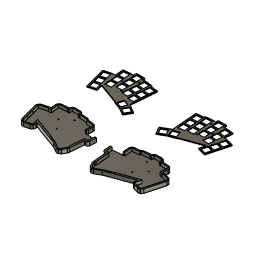
Architeuthis Dux v2 (Autodesk Fusion 360 design; units mm, degrees)
Autodesk Fusion 360 part; units mm, degrees
note: some values were not read from the file. Set by a fixed rule: which sketch regions a step uses.
sketch "Sketch1" plane through (0, 0, 0) normal (0, 0, 1) x (1, 0, 0)
  line L0 (25.9385, -60.9067) -> (30.3403, -77.3278)
  line L1 (30.3403, -77.3278) -> (12.954, -81.9861)
  line L2 (12.954, -81.9861) -> (8.5522, -65.565)
  line L3 (21.5392, -44.4856) -> (25.9385, -60.9067)
  line L4 (25.9385, -60.9067) -> (8.5522, -65.565)
  line L5 (25.9385, -60.9067) -> (8.5522, -65.565)
  line L6 (8.5522, -65.565) -> (4.1529, -49.1439)
  line L7 (4.1529, -49.1439) -> (21.5392, -44.4856)
  line L8 (-0.2438, -32.7228) -> (17.1399, -28.0645)
  line L9 (17.1399, -28.0645) -> (21.5392, -44.4856)
  line L10 (4.1529, -49.1439) -> (-0.2438, -32.7228)
  line L11 (43.5762, -40.5994) -> (45.0571, -57.5361)
  line L12 (45.0571, -57.5361) -> (27.1272, -59.1033)
  line L13 (27.1272, -59.1033) -> (25.6438, -42.1691)
  line L14 (25.6438, -42.1691) -> (43.5762, -40.5994)
  line L15 (43.5762, -40.5994) -> (25.6438, -42.1691)
  line L16 (43.5762, -40.5994) -> (25.6438, -42.1691)
  line L17 (25.6438, -42.1691) -> (24.163, -25.2349)
  line L18 (24.163, -25.2349) -> (42.0954, -23.6652)
  line L19 (42.0954, -23.6652) -> (43.5762, -40.5994)
  line L20 (24.163, -25.2349) -> (22.6822, -8.2982)
  line L21 (22.6822, -8.2982) -> (40.6121, -6.7285)
  line L22 (40.6121, -6.7285) -> (42.0954, -23.6652)
  line L23 (45.4711, -34.0741) -> (63.4695, -34.0741)
  line L24 (63.4695, -34.0741) -> (63.4695, -51.0743)
  line L25 (63.4695, -51.0743) -> (45.4711, -51.0743)
  line L26 (45.4711, -51.0743) -> (45.4711, -34.0741)
  line L27 (45.4711, -34.0741) -> (63.4695, -34.0741)
  line L28 (45.4711, -17.0739) -> (63.4695, -17.0739)
  line L29 (45.4711, -34.0741) -> (45.4711, -17.0739)
  line L30 (63.4695, -34.0741) -> (45.4711, -34.0741)
  line L31 (63.4695, -17.0739) -> (63.4695, -34.0741)
  line L32 (63.4695, -0.0737) -> (63.4695, -17.0739)
  line L33 (45.4711, -17.0739) -> (45.4711, -0.0737)
  line L34 (45.4711, -0.0737) -> (63.4695, -0.0737)
  line L35 (65.5269, -39.0525) -> (83.4593, -40.6222)
  line L36 (83.4593, -40.6222) -> (81.976, -57.5564)
  line L37 (81.976, -57.5564) -> (64.0461, -55.9892)
  line L38 (64.0461, -55.9892) -> (65.5269, -39.0525)
  line L39 (65.5269, -39.0525) -> (83.4593, -40.6222)
  line L40 (67.0077, -22.1183) -> (84.9401, -23.6855)
  line L41 (65.5269, -39.0525) -> (67.0077, -22.1183)
  line L42 (86.421, -6.7513) -> (84.9401, -23.6855)
  line L43 (67.0077, -22.1183) -> (68.4911, -5.1816)
  line L44 (68.4911, -5.1816) -> (86.421, -6.7513)
  line L45 (83.2129, -43.4442) -> (101.1428, -45.0139)
  line L46 (101.1428, -45.0139) -> (99.662, -61.9481)
  line L47 (99.662, -61.9481) -> (81.7296, -60.3809)
  line L48 (81.7296, -60.3809) -> (83.2129, -43.4442)
  line L49 (83.2129, -43.4442) -> (101.1428, -45.0139)
  line L50 (84.6938, -26.51) -> (102.6262, -28.0772)
  line L51 (102.6262, -28.0772) -> (101.1428, -45.0139)
  line L52 (86.1746, -9.5733) -> (104.107, -11.143)
  line L53 (102.6262, -28.0772) -> (84.6938, -26.51)
  line L54 (104.107, -11.143) -> (102.6262, -28.0772)
  line L55 (83.7946, -65.5396) -> (100.7085, -71.6966)
  line L56 (94.8944, -87.6706) -> (77.9805, -81.5137)
  line L57 (77.9805, -81.5137) -> (83.7946, -65.5396)
  line L58 (100.7085, -71.6966) -> (94.8944, -87.6706)
  line L59 (103.5533, -73.0225) -> (119.1412, -82.0217)
  line L60 (119.1412, -82.0217) -> (110.6424, -96.7435)
  line L61 (110.6424, -96.7435) -> (95.0519, -87.7443)
  line L62 (95.0519, -87.7443) -> (103.5533, -73.0225)
  line L63 (116.5835, -26.9875) -> (116.1415, -32.0472)
  line L64 (108.9914, -26.322) -> (116.5835, -26.9875)
  line L65 (108.5494, -31.3817) -> (108.9914, -26.322)
  line L66 (116.1415, -32.0472) -> (108.5494, -31.3817)
  line L67 (128.7755, -30.3657) -> (123.1951, -29.878)
  line L68 (123.0224, -31.8694) -> (123.1951, -29.878)
  line L69 (128.6002, -32.3571) -> (128.7755, -30.3657)
  line L70 (122.7734, -31.8491) -> (121.7193, -43.9014)
  line L71 (128.8491, -32.3799) -> (127.795, -44.4348)
  line L72 (127.795, -44.4348) -> (121.7193, -43.9014)
  line L73 (128.8491, -32.3799) -> (122.7734, -31.8491)
  arc A0 (94.8962, -87.6719) -> (95.0542, -87.7456) centre (94.5542, -88.6116) cw
  line L74 (83.4593, -40.6222) -> (84.9401, -23.6855)
  line L75 (84.6938, -26.51) -> (86.1746, -9.5733)
  line L76 (83.2129, -43.4442) -> (84.6938, -26.51)
  line L77 (2.0726, -33.655) -> (5.6972, -47.178)
  line L78 (5.6972, -47.178) -> (19.2202, -43.5559)
  line L79 (19.2202, -43.5559) -> (15.5956, -30.033)
  line L80 (15.5956, -30.033) -> (2.0726, -33.655)
  line L81 (6.4719, -50.0761) -> (10.0965, -63.5991)
  line L82 (10.0965, -63.5991) -> (23.6195, -59.9745)
  line L83 (23.6195, -59.9745) -> (19.9949, -46.4515)
  line L84 (19.9949, -46.4515) -> (6.4719, -50.0761)
  line L85 (10.8737, -66.4972) -> (14.4958, -80.0202)
  line L86 (14.4958, -80.0202) -> (28.0187, -76.3956)
  line L87 (28.0187, -76.3956) -> (24.3967, -62.8726)
  line L88 (24.3967, -62.8726) -> (10.8737, -66.4972)
  line L89 (27.7673, -43.4899) -> (28.989, -57.437)
  line L90 (28.989, -57.437) -> (42.9336, -56.2153)
  line L91 (42.9336, -56.2153) -> (41.7144, -42.2681)
  line L92 (41.7144, -42.2681) -> (27.7673, -43.4899)
  line L93 (26.2865, -26.5532) -> (27.5057, -40.5003)
  line L94 (27.5057, -40.5003) -> (41.4528, -39.2811)
  line L95 (41.4528, -39.2811) -> (40.2336, -25.334)
  line L96 (40.2336, -25.334) -> (26.2865, -26.5532)
  line L97 (24.8056, -9.619) -> (26.0248, -23.5661)
  line L98 (26.0248, -23.5661) -> (39.972, -22.3444)
  line L99 (39.972, -22.3444) -> (38.7502, -8.3972)
  line L100 (38.7502, -8.3972) -> (24.8056, -9.619)
  line L101 (47.4701, -1.5748) -> (47.4701, -15.5727)
  line L102 (47.4701, -15.5727) -> (61.4705, -15.5727)
  line L103 (61.4705, -15.5727) -> (61.4705, -1.5748)
  line L104 (61.4705, -1.5748) -> (47.4701, -1.5748)
  line L105 (47.4701, -18.5725) -> (47.4701, -32.573)
  line L106 (47.4701, -32.573) -> (61.4705, -32.573)
  line L107 (61.4705, -32.573) -> (61.4705, -18.5725)
  line L108 (61.4705, -18.5725) -> (47.4701, -18.5725)
  line L109 (47.4701, -35.5727) -> (47.4701, -49.5732)
  line L110 (47.4701, -49.5732) -> (61.4705, -49.5732)
  line L111 (61.4705, -49.5732) -> (61.4705, -35.5727)
  line L112 (61.4705, -35.5727) -> (47.4701, -35.5727)
  line L113 (67.3887, -40.7213) -> (66.1695, -54.6684)
  line L114 (66.1695, -54.6684) -> (80.1141, -55.8876)
  line L115 (80.1141, -55.8876) -> (81.3359, -41.943)
  line L116 (81.3359, -41.943) -> (67.3887, -40.7213)
  line L117 (68.8696, -23.7871) -> (67.6504, -37.7342)
  line L118 (67.6504, -37.7342) -> (81.5975, -38.9534)
  line L119 (81.5975, -38.9534) -> (82.8167, -25.0063)
  line L120 (82.8167, -25.0063) -> (68.8696, -23.7871)
  line L121 (70.3529, -6.8504) -> (69.1312, -20.7975)
  line L122 (69.1312, -20.7975) -> (83.0783, -22.0167)
  line L123 (83.0783, -22.0167) -> (84.3001, -8.0721)
  line L124 (84.3001, -8.0721) -> (70.3529, -6.8504)
  line L125 (88.0364, -11.242) -> (86.8172, -25.1892)
  line L126 (86.8172, -25.1892) -> (100.7643, -26.4084)
  line L127 (100.7643, -26.4084) -> (101.9835, -12.4638)
  line L128 (101.9835, -12.4638) -> (88.0364, -11.242)
  line L129 (86.5556, -28.1788) -> (85.3338, -42.1234)
  line L130 (85.3338, -42.1234) -> (99.281, -43.3451)
  line L131 (99.281, -43.3451) -> (100.5027, -29.398)
  line L132 (100.5027, -29.398) -> (86.5556, -28.1788)
  line L133 (85.0722, -45.1129) -> (83.853, -59.0601)
  line L134 (83.853, -59.0601) -> (97.8002, -60.2793)
  line L135 (97.8002, -60.2793) -> (99.0194, -46.3321)
  line L136 (99.0194, -46.3321) -> (85.0722, -45.1129)
  line L137 (85.1611, -67.6326) -> (80.3732, -80.7898)
  line L138 (80.3732, -80.7898) -> (93.5279, -85.5777)
  line L139 (93.5279, -85.5777) -> (98.3158, -72.4205)
  line L140 (98.3158, -72.4205) -> (85.1611, -67.6326)
  line L141 (104.5337, -75.3212) -> (97.536, -87.4446)
  line L142 (97.536, -87.4446) -> (109.6594, -94.4448)
  line L143 (109.6594, -94.4448) -> (116.6597, -82.3214)
  line L144 (116.6597, -82.3214) -> (104.5337, -75.3212)
  line L145 (3.1869, -49.4026) -> (-1.4684, -32.0157)
  line L146 (-1.4684, -32.0157) -> (17.8471, -26.8397)
  line L147 (17.8471, -26.8397) -> (22.5051, -44.2268)
  line L148 (22.5051, -44.2268) -> (26.9044, -60.6478)
  line L149 (26.9044, -60.6478) -> (31.5651, -78.0349)
  line L150 (31.5651, -78.0349) -> (12.247, -83.2108)
  line L151 (12.247, -83.2108) -> (7.5863, -65.8239)
  line L152 (7.5863, -65.8239) -> (3.1869, -49.4026)
  line L153 (23.2539, -26.3183) -> (21.5989, -7.3892)
  line L154 (21.5989, -7.3892) -> (41.521, -5.6451)
  line L155 (41.521, -5.6451) -> (43.1789, -24.5742)
  line L156 (23.2539, -26.3183) -> (43.1789, -24.5742)
  line L157 (44.4711, -18.0739) -> (44.4711, 0.9263)
  line L158 (44.4711, 0.9263) -> (64.4695, 0.9263)
  line L159 (64.4695, 0.9263) -> (64.4695, -18.0739)
  line L160 (44.4711, -18.0739) -> (64.4695, -18.0739)
  line L161 (65.9243, -23.0274) -> (67.5822, -4.0982)
  line L162 (67.5822, -4.0982) -> (87.5043, -5.8423)
  line L163 (87.5043, -5.8423) -> (85.8492, -24.7688)
  line L164 (65.9243, -23.0274) -> (85.8492, -24.7688)
  line L165 (83.6105, -27.4191) -> (85.2655, -8.4899)
  line L166 (85.2655, -8.4899) -> (105.1903, -10.234)
  line L167 (105.1903, -10.234) -> (103.5352, -29.1604)
  line L168 (103.5352, -29.1604) -> (83.6105, -27.4191)
  line L169 (76.6988, -82.1113) -> (83.1969, -64.2579)
  line L170 (83.1969, -64.2579) -> (101.9902, -71.0989)
  line L171 (101.9902, -71.0989) -> (95.4921, -88.9524)
  line L172 (95.4921, -88.9524) -> (76.6988, -82.1113)
  line L173 (120.5072, -81.6556) -> (111.0085, -98.1095)
  line L174 (111.0085, -98.1095) -> (93.6857, -88.1104)
  line L175 (93.6857, -88.1104) -> (103.1873, -71.6565)
  line L176 (103.1873, -71.6565) -> (120.5072, -81.6556)
  point P0 (104.5337, -75.3212)
  point P1 (97.536, -87.4446)
  point P2 (109.6594, -94.4448)
  point P3 (116.6597, -82.3214)
  point P4 (93.5279, -85.5777)
  point P5 (98.3158, -72.4205)
  point P6 (85.1611, -67.6326)
  point P7 (80.3732, -80.7898)
  point P8 (97.8002, -60.2793)
  point P9 (99.0194, -46.3321)
  point P10 (85.0722, -45.1129)
  point P11 (83.853, -59.0601)
  point P12 (85.3338, -42.1234)
  point P13 (99.281, -43.3451)
  point P14 (100.5027, -29.398)
  point P15 (86.5556, -28.1788)
  point P16 (86.8172, -25.1892)
  point P17 (88.0364, -11.242)
  point P18 (101.9835, -12.4638)
  point P19 (100.7643, -26.4084)
  point P20 (83.0783, -22.0167)
  point P21 (84.3001, -8.0721)
  point P22 (70.3529, -6.8504)
  point P23 (69.1312, -20.7975)
  point P24 (68.8696, -23.7871)
  point P25 (82.8167, -25.0063)
  point P26 (81.5975, -38.9534)
  point P27 (67.6504, -37.7342)
  point P28 (67.3887, -40.7213)
  point P29 (81.3359, -41.943)
  point P30 (80.1141, -55.8876)
  point P31 (66.1695, -54.6684)
  point P32 (61.4705, -49.5732)
  point P33 (61.4705, -35.5727)
  point P34 (47.4701, -35.5727)
  point P35 (47.4701, -49.5732)
  point P36 (47.4701, -32.573)
  point P37 (61.4705, -32.573)
  point P38 (61.4705, -18.5725)
  point P39 (47.4701, -18.5725)
  point P40 (47.4701, -15.5727)
  point P41 (61.4705, -15.5727)
  point P42 (61.4705, -1.5748)
  point P43 (47.4701, -1.5748)
  point P44 (38.7502, -8.3972)
  point P45 (24.8056, -9.619)
  point P46 (26.0248, -23.5661)
  point P47 (39.972, -22.3444)
  point P48 (40.2336, -25.334)
  point P49 (26.2865, -26.5532)
  point P50 (41.4528, -39.2811)
  point P51 (27.5057, -40.5003)
  point P52 (27.7673, -43.4899)
  point P53 (41.7144, -42.2681)
  point P54 (42.9336, -56.2153)
  point P55 (28.989, -57.437)
  point P56 (15.5956, -30.033)
  point P57 (2.0726, -33.655)
  point P58 (19.2202, -43.5559)
  point P59 (5.6972, -47.178)
  point P60 (6.4719, -50.0761)
  point P61 (19.9949, -46.4515)
  point P62 (23.6195, -59.9745)
  point P63 (10.0965, -63.5991)
  point P64 (24.3967, -62.8726)
  point P65 (28.0187, -76.3956)
  point P66 (14.4958, -80.0202)
  point P67 (10.8737, -66.4972)
  dimension "d8" = -1
  dimension "d9" = 1
  dimension "d10" = 1
  dimension "d11" = 1
  dimension "d12" = -1
  dimension "d13" = -1
  dimension "d14" = -1
  constraint coincident P57 L77.start
  constraint coincident P59 L77.end
  constraint coincident P58 L78.end
  constraint coincident P56 L79.end
  constraint parallel L77 L79
  constraint parallel L78 L80
  constraint coincident P60 L81.start
  constraint coincident P63 L81.end
  constraint parallel L77 L81
  constraint coincident P62 L82.end
  constraint perpendicular L81 L82
  constraint coincident P61 L83.end
  constraint parallel L81 L83
  constraint perpendicular L81 L84
  constraint coincident P67 L85.start
  constraint coincident P66 L85.end
  constraint coincident P65 L86.end
  constraint parallel L82 L86
  constraint coincident P64 L87.end
  constraint parallel L85 L87
  constraint coincident P52 L89.start
  constraint coincident P55 L89.end
  constraint coincident P54 L90.end
  constraint coincident P53 L91.end
  constraint perpendicular L89 L92
  constraint coincident P49 L93.start
  constraint coincident P51 L93.end
  constraint coincident P50 L94.end
  constraint coincident P48 L95.end
  constraint coincident P45 L97.start
  constraint coincident P46 L97.end
  constraint parallel L93 L97
  constraint coincident P47 L98.end
  constraint coincident P44 L99.end
  constraint perpendicular L98 L99
  constraint coincident P43 L101.start
  constraint coincident P40 L101.end
  constraint parallel L33 L101
  constraint coincident P41 L102.end
  constraint perpendicular L101 L102
  constraint coincident P42 L103.end
  constraint perpendicular L102 L103
  constraint perpendicular L101 L104
  constraint coincident P39 L105.start
  constraint coincident P36 L105.end
  constraint perpendicular L28 L105
  constraint coincident P37 L106.end
  constraint perpendicular L105 L106
  constraint coincident P38 L107.end
  constraint perpendicular L106 L107
  constraint perpendicular L107 L108
  constraint coincident P34 L109.start
  constraint coincident P35 L109.end
  constraint perpendicular L106 L109
  constraint coincident P32 L110.end
  constraint perpendicular L109 L110
  constraint coincident P33 L111.end
  constraint perpendicular L106 L111
  constraint perpendicular L109 L112
  constraint coincident P28 L113.start
  constraint coincident P31 L113.end
  constraint coincident P30 L114.end
  constraint coincident P29 L115.end
  constraint coincident P24 L117.start
  constraint coincident P27 L117.end
  constraint coincident P26 L118.end
  constraint perpendicular L117 L118
  constraint coincident P25 L119.end
  constraint perpendicular L118 L119
  constraint perpendicular L117 L120
  constraint coincident P22 L121.start
  constraint coincident P23 L121.end
  constraint coincident P20 L122.end
  constraint coincident P21 L123.end
  constraint coincident P17 L125.start
  constraint coincident P16 L125.end
  constraint coincident P19 L126.end
  constraint perpendicular L125 L126
  constraint coincident P18 L127.end
  constraint coincident P15 L129.start
  constraint coincident P12 L129.end
  constraint coincident P13 L130.end
  constraint parallel L128 L130
  constraint coincident P14 L131.end
  constraint perpendicular L130 L131
  constraint coincident P10 L133.start
  constraint coincident P11 L133.end
  constraint coincident P8 L134.end
  constraint perpendicular L133 L134
  constraint coincident P9 L135.end
  constraint perpendicular L134 L135
  constraint perpendicular L135 L136
  constraint coincident P6 L137.start
  constraint coincident P7 L137.end
  constraint coincident P4 L138.end
  constraint coincident P5 L139.end
  constraint parallel L137 L139
  constraint parallel L138 L140
  constraint coincident P0 L141.start
  constraint coincident P1 L141.end
  constraint coincident P2 L142.end
  constraint coincident P3 L143.end
  constraint perpendicular L142 L143
sketch "Sketch2" plane through (0, 0, 0) normal (0, 0, 1) x (1, 0, 0)
  arc A0 (12.963, -80.5576) -> (11.5653, -78.7359) centre (14.463, -77.9596) cw
  arc A1 (29.9179, -73.8185) -> (29.6182, -76.0948) centre (27.0201, -74.5949) cw
  arc A2 (29.2646, -76.7072) -> (27.4429, -78.105) centre (26.6666, -75.2072) cw
  arc A3 (15.8519, -81.2109) -> (13.5754, -80.9112) centre (15.0754, -78.3131) cw
  arc A4 (0.1772, -36.2354) -> (0.4769, -33.9588) centre (3.075, -35.4588) cw
  arc A5 (0.8305, -33.3464) -> (2.6521, -31.9486) centre (3.4285, -34.8464) cw
  arc A6 (22.4896, -11.83) -> (23.18, -9.6402) centre (25.4781, -11.5685) cw
  arc A7 (23.6345, -9.0985) -> (25.6713, -8.0383) centre (25.9326, -11.0268) cw
  arc A8 (44.9717, -3.575) -> (45.8506, -1.4537) centre (47.9717, -3.5752) cw
  arc A9 (46.3504, -0.9537) -> (48.4718, -0.075) centre (48.4717, -3.075) cw
  arc A10 (60.4718, -0.075) -> (62.593, -0.9537) centre (60.4716, -3.075) cw
  arc A11 (63.0931, -1.4537) -> (63.9717, -3.575) centre (60.9717, -3.5749) cw
  arc A12 (83.4347, -6.491) -> (85.4713, -7.5512) centre (83.1731, -9.4796) cw
  arc A13 (85.9259, -8.0929) -> (86.4535, -9.0137) centre (83.6277, -10.0212) cw
  arc A14 (101.1192, -10.8824) -> (103.156, -11.9426) centre (100.8579, -13.871) cw
  arc A15 (103.6104, -12.4843) -> (104.3008, -14.6741) centre (101.3122, -14.4126) cw
  arc A16 (118.2164, -83.5449) -> (117.8258, -85.3044) centre (115.2277, -83.8044) cw
  arc A17 (112.8258, -93.9645) -> (111.0041, -95.3623) centre (110.2277, -92.4645) cw
  arc A18 (110.3211, -95.5454) -> (108.0447, -95.2457) centre (109.5447, -92.6476) cw
  arc A19 (23.6819, -25.4584) -> (22.9445, -26.5115) centre (22.6857, -25.5456) cw
  arc A20 (44.9717, -5.4333) -> (44.0588, -6.4296) centre (43.9717, -5.4334) cw
  arc A21 (64.8846, -4.8681) -> (63.9717, -3.8719) centre (64.9717, -3.8719) cw
  arc A22 (87.3082, -9.6741) -> (86.4535, -9.0137) centre (87.3954, -8.6779) cw
  arc A23 (104.1204, -28.21) -> (103.2114, -27.1264) centre (104.2075, -27.2138) cw
  arc A24 (129.0254, -30.3888) -> (129.9345, -31.4721) centre (128.9383, -31.385) cw
  arc A25 (128.6271, -46.4149) -> (127.5438, -47.324) centre (127.6309, -46.3278) cw
  arc A26 (121.33, -47.7843) -> (122.4133, -46.8752) centre (122.3262, -47.8714) cw
  arc A27 (94.8962, -87.6719) -> (95.0542, -87.7456) centre (94.5542, -88.6116) cw
  arc A28 (27.5064, -64.8185) -> (28.8143, -63.6201) centre (28.4724, -64.5599) cw
  line L0 (29.6182, -76.0948) -> (29.2646, -76.7072)
  line L1 (29.9179, -73.8185) -> (27.5064, -64.8185)
  line L2 (28.8143, -63.6201) -> (94.8962, -87.6719)
  line L3 (95.0542, -87.7456) -> (108.0447, -95.2457)
  line L4 (110.3211, -95.5454) -> (111.0041, -95.3623)
  line L5 (112.8258, -93.9645) -> (117.8258, -85.3044)
  line L6 (118.2164, -83.3712) -> (121.33, -47.7843)
  line L7 (122.4133, -46.8752) -> (127.5438, -47.324)
  line L8 (128.6271, -46.4149) -> (129.9345, -31.4721)
  line L9 (129.0254, -30.3888) -> (104.1204, -28.21)
  line L10 (103.2114, -27.1264) -> (104.3008, -14.6741)
  line L11 (87.3082, -9.6741) -> (101.1192, -10.8824)
  line L12 (64.8846, -4.8681) -> (83.4347, -6.491)
  line L13 (48.4718, -0.075) -> (60.4718, -0.075)
  line L14 (44.9717, -3.575) -> (44.9717, -5.4333)
  line L15 (25.6713, -8.0383) -> (44.0588, -6.4296)
  line L16 (22.4896, -11.83) -> (23.6819, -25.4584)
  line L17 (2.6521, -31.9486) -> (22.9445, -26.5115)
  line L18 (0.1772, -36.2354) -> (11.5653, -78.7359)
  line L19 (15.8519, -81.2109) -> (27.4429, -78.105)
  line L20 (118.2164, -83.5449) -> (118.2164, -83.3712)
  line L21 (103.156, -11.9426) -> (103.6104, -12.4843)
  line L22 (85.4713, -7.5512) -> (85.9259, -8.0929)
  line L23 (63.9717, -3.8719) -> (63.9717, -3.575)
  line L24 (62.593, -0.9537) -> (63.0931, -1.4537)
  line L25 (45.8506, -1.4537) -> (46.3504, -0.9537)
  line L26 (23.18, -9.6402) -> (23.6345, -9.0985)
  line L27 (0.4769, -33.9588) -> (0.8305, -33.3464)
  line L28 (12.963, -80.5576) -> (13.5754, -80.9112)
  line L29 (25.3225, -4.0535) -> (41.0293, -2.6793)
  arc A29 (25.3225, -4.0535) -> (20.5703, -6.5274) centre (25.9326, -11.0268) ccw
  line L30 (20.1158, -7.0691) -> (20.5703, -6.5274)
  arc A30 (20.1158, -7.0691) -> (18.5048, -12.1786) centre (25.4781, -11.5685) ccw
  line L31 (18.5048, -12.1786) -> (19.4777, -23.2993)
  line L32 (1.6168, -28.0849) -> (19.4777, -23.2993)
  arc A31 (1.6168, -28.0849) -> (-2.6337, -31.3465) centre (3.4285, -34.8464) ccw
  line L33 (-2.9872, -31.9588) -> (-2.6337, -31.3465)
  arc A32 (-2.9872, -31.9588) -> (-3.6865, -37.2707) centre (3.075, -35.4588) ccw
  line L34 (-3.6865, -37.2707) -> (7.7016, -79.7712)
  arc A33 (7.7016, -79.7712) -> (10.963, -84.0217) centre (14.463, -77.9596) ccw
  line L35 (10.963, -84.0217) -> (11.5753, -84.3753)
  arc A34 (11.5753, -84.3753) -> (16.8872, -85.0746) centre (15.0754, -78.3131) ccw
  line L36 (16.8872, -85.0746) -> (28.4782, -81.9687)
  arc A35 (28.4782, -81.9687) -> (32.7287, -78.7072) centre (26.6666, -75.2072) ccw
  line L37 (33.0822, -78.0949) -> (32.7287, -78.7072)
  arc A36 (33.0822, -78.0949) -> (33.7816, -72.7832) centre (27.0201, -74.5949) ccw
  line L38 (33.7816, -72.7832) -> (32.8617, -69.35)
  line L39 (32.8617, -69.35) -> (93.2815, -91.3409)
  line L40 (93.2815, -91.3409) -> (106.0447, -98.7098)
  arc A37 (106.0447, -98.7098) -> (111.3571, -99.4089) centre (109.5447, -92.6476) ccw
  line L41 (111.3571, -99.4089) -> (112.0401, -99.2258)
  arc A38 (112.0401, -99.2258) -> (116.2899, -95.9645) centre (110.2277, -92.4645) ccw
  line L42 (116.2899, -95.9645) -> (121.2898, -87.3045)
  arc A39 (121.2898, -87.3045) -> (122.2208, -83.4953) centre (115.2277, -83.8044) ccw
  line L43 (122.2208, -83.4953) -> (125.0533, -51.1214)
  line L44 (125.0533, -51.1214) -> (127.1953, -51.3088)
  arc A40 (127.1953, -51.3088) -> (132.6119, -46.7636) centre (127.6309, -46.3278) ccw
  line L45 (132.6119, -46.7636) -> (133.9192, -31.8207)
  arc A41 (133.9192, -31.8207) -> (129.374, -26.404) centre (128.9383, -31.385) ccw
  line L46 (129.374, -26.404) -> (107.4576, -24.4867)
  line L47 (107.4576, -24.4867) -> (108.2856, -15.0227)
  arc A42 (108.2856, -15.0227) -> (106.6753, -9.9139) centre (101.3122, -14.4126) ccw
  line L48 (106.2206, -9.3719) -> (106.6753, -9.9139)
  arc A43 (106.2206, -9.3719) -> (101.4678, -6.8976) centre (100.8579, -13.871) ccw
  line L49 (89.2321, -5.8271) -> (101.4678, -6.8976)
  arc A44 (89.2321, -5.8271) -> (88.989, -5.5205) centre (83.6277, -10.0212) ccw
  line L50 (88.5345, -4.979) -> (88.989, -5.5205)
  arc A45 (88.5345, -4.979) -> (83.7831, -2.5062) centre (83.1731, -9.4796) ccw
  line L51 (67.513, -1.0828) -> (83.7831, -2.5062)
  arc A46 (67.513, -1.0828) -> (65.9211, 1.3752) centre (60.9717, -3.5749) ccw
  line L52 (65.4205, 1.8756) -> (65.9211, 1.3752)
  arc A47 (65.4205, 1.8756) -> (60.4715, 3.925) centre (60.4716, -3.075) ccw
  line L53 (48.4717, 3.925) -> (60.4715, 3.925)
  arc A48 (48.4717, 3.925) -> (43.5211, 1.8739) centre (48.4717, -3.075) ccw
  line L54 (43.0217, 1.3743) -> (43.5211, 1.8739)
  arc A49 (43.0217, 1.3743) -> (41.0293, -2.6793) centre (47.9717, -3.5752) ccw
  dimension "d1" = -4
  constraint tangent A2 L0
  constraint tangent A18 L3
  constraint tangent A26 L6
  constraint tangent A25 L7
  constraint tangent A15 L10
  constraint tangent A20 L14
  constraint tangent A20 L15
  constraint tangent A19 L16
  constraint tangent A19 L17
  constraint tangent A7 L26
  constraint tangent A5 L27
extrude "Extrude1" add sketch "Sketch2" against normal blind 2 contours A0 A1 A2 A3 A4 A5 A6 A7 A8 A9 A10 A11 A12 A13 A14 A15 A16 A17 A18 A19 A20 A21 A22 A23 A24 A25 A26 A27 A28 L0 L1 L2 L3 L4 L5 L6 L7 L8 L9 L10 L11 L12 L13 L14 L15 L16 L17 L18 L19 L20 L21 L22 L23 L24 L25 L26 L27 L28 makes body 1
extrude "Extrude2" add sketch "Sketch2" along normal blind 7 and the other way blind 2 bodies 1
extrude "Extrude3" cut sketch "Sketch1" along normal blind 7 contours L0 L1 L2 L4 L5 | L7 L8 L9 L10 | L17 L19 L20 L21 L22 L153 L154 L155 L156 | L18 L20 L21 L22 | L29 L31 L32 L33 L34 L157 L158 L159 L160 | L28 L32 L33 L34 | L41 L42 L43 L44 L161 L162 L163 L164 L166 | L40 L42 L43 L44 L165 L166 | L50 L52 L53 L54 L74 L75 L163 L164 | L51 L52 L54 L163 L166 L167 L168 | L40 L42 L75 L165 L166 | L42 L52 L74 L75 L163 L164 | L42 L52 L163 L166 | L55 L56 L57 L58 L169 L170 L171 L172 L174 L175 | L58 L62 A0 L171 L175 | L56 L58 L175 | L56 L61 A0 L171 L172 L174 L175 | L59 L60 L61 L62 L171 L172 L173 L174 L175 L176 | L61 L62 A0 L171 | L59 L60 L61 L62 L171 | L145 L146 L147 L148 L149 L150 L151 L152 bodies 1
sketch "Sketch3" plane through (0, 0, 7) normal (0, 0, 1) x (-1, 0, 0)
  line L0 (-64.4695, -0.9263) -> (-64.4695, 4.7367)
  arc A0 (-64.4695, 4.7367) -> (-64.8846, 4.8681) centre (-64.9717, 3.8719) ccw
  line L1 (-64.8846, 4.8681) -> (-67.4947, 5.0964)
  line L2 (-67.4947, 5.0964) -> (-67.5822, 4.0982)
  line L3 (-67.5822, 4.0982) -> (-87.5043, 5.8423)
  line L4 (-87.5043, 5.8423) -> (-87.2575, 8.6642)
  line L5 (-87.2575, 8.6642) -> (-105.1903, 10.234)
  line L6 (-105.1903, 10.234) -> (-103.6338, 28.0329)
  arc A1 (-103.6338, 28.0329) -> (-104.1204, 28.21) centre (-104.2075, 27.2138) ccw
  line L7 (-104.1204, 28.21) -> (-129.0254, 30.3888)
  arc A2 (-129.9345, 31.4721) -> (-129.0254, 30.3888) centre (-128.9383, 31.385) ccw
  line L8 (-129.9345, 31.4721) -> (-128.6271, 46.4149)
  arc A3 (-127.5438, 47.324) -> (-128.6271, 46.4149) centre (-127.6309, 46.3278) ccw
  line L9 (-127.5438, 47.324) -> (-122.4133, 46.8752)
  arc A4 (-122.4133, 46.8752) -> (-121.33, 47.7843) centre (-122.3262, 47.8714) ccw
  line L10 (-121.33, 47.7843) -> (-118.4694, 80.4792)
  line L11 (-118.4694, 80.4792) -> (-120.5072, 81.6556)
  line L12 (-120.5072, 81.6556) -> (-111.0085, 98.1095)
  line L13 (-111.0085, 98.1095) -> (-94.5511, 88.6099)
  line L14 (-94.5511, 88.6099) -> (-76.6988, 82.1113)
  line L15 (-76.6988, 82.1113) -> (-77.0404, 81.173)
  line L16 (-77.0404, 81.173) -> (-28.8143, 63.6201)
  arc A5 (-28.8143, 63.6201) -> (-27.7639, 63.8542) centre (-28.4724, 64.5599) ccw
  line L17 (-27.7639, 63.8542) -> (-31.5651, 78.0349)
  line L18 (-31.5651, 78.0349) -> (-12.247, 83.2108)
  line L19 (-12.247, 83.2108) -> (-7.5863, 65.8239)
  line L20 (-7.5863, 65.8239) -> (-3.1869, 49.4026)
  line L21 (-3.1869, 49.4026) -> (1.4684, 32.0157)
  line L22 (1.4684, 32.0157) -> (-17.8471, 26.8397)
  line L23 (-17.8471, 26.8397) -> (-18.1064, 27.8078)
  line L24 (-18.1064, 27.8078) -> (-22.9445, 26.5115)
  arc A6 (-22.9445, 26.5115) -> (-23.3283, 26.3118) centre (-22.6857, 25.5456) ccw
  line L25 (-23.3283, 26.3118) -> (-23.2539, 26.3183)
  line L26 (-23.2539, 26.3183) -> (-21.5989, 7.3892)
  line L27 (-21.5989, 7.3892) -> (-41.521, 5.6451)
  line L28 (-41.521, 5.6451) -> (-41.6085, 6.6439)
  line L29 (-41.6085, 6.6439) -> (-44.0588, 6.4296)
  arc A7 (-44.0588, 6.4296) -> (-44.4711, 6.2997) centre (-43.9717, 5.4334) ccw
  line L30 (-44.4711, 6.2997) -> (-44.4711, -0.9263)
  line L31 (-44.4711, -0.9263) -> (-64.4695, -0.9263)
  arc A8 (-48.4717, -3.925) -> (-43.5211, -1.8739) centre (-48.4717, 3.075) ccw
  line L32 (-43.5211, -1.8739) -> (-43.0217, -1.3743)
  arc A9 (-43.0217, -1.3743) -> (-41.0293, 2.6793) centre (-47.9717, 3.5752) ccw
  line L33 (-41.0293, 2.6793) -> (-25.3225, 4.0535)
  arc A10 (-25.3225, 4.0535) -> (-20.5703, 6.5274) centre (-25.9326, 11.0268) ccw
  line L34 (-20.5703, 6.5274) -> (-20.1158, 7.0691)
  arc A11 (-20.1158, 7.0691) -> (-18.5048, 12.1786) centre (-25.4781, 11.5685) ccw
  line L35 (-18.5048, 12.1786) -> (-19.4777, 23.2993)
  line L36 (-19.4777, 23.2993) -> (-1.6168, 28.0849)
  arc A12 (-1.6168, 28.0849) -> (2.6337, 31.3465) centre (-3.4285, 34.8464) ccw
  line L37 (2.6337, 31.3465) -> (2.9872, 31.9588)
  arc A13 (2.9872, 31.9588) -> (3.6865, 37.2707) centre (-3.075, 35.4588) ccw
  line L38 (3.6865, 37.2707) -> (-7.7016, 79.7712)
  arc A14 (-7.7016, 79.7712) -> (-10.963, 84.0217) centre (-14.463, 77.9596) ccw
  line L39 (-10.963, 84.0217) -> (-11.5753, 84.3753)
  arc A15 (-11.5753, 84.3753) -> (-16.8872, 85.0746) centre (-15.0754, 78.3131) ccw
  line L40 (-16.8872, 85.0746) -> (-28.4782, 81.9687)
  arc A16 (-28.4782, 81.9687) -> (-32.7287, 78.7072) centre (-26.6666, 75.2072) ccw
  line L41 (-32.7287, 78.7072) -> (-33.0822, 78.0949)
  arc A17 (-33.0822, 78.0949) -> (-33.7816, 72.7832) centre (-27.0201, 74.5949) ccw
  line L42 (-33.7816, 72.7832) -> (-32.8617, 69.35)
  line L43 (-32.8617, 69.35) -> (-93.2815, 91.3409)
  line L44 (-93.2815, 91.3409) -> (-106.0447, 98.7098)
  arc A18 (-106.0447, 98.7098) -> (-111.3571, 99.4089) centre (-109.5447, 92.6476) ccw
  line L45 (-111.3571, 99.4089) -> (-112.0401, 99.2258)
  arc A19 (-112.0401, 99.2258) -> (-116.2899, 95.9645) centre (-110.2277, 92.4645) ccw
  line L46 (-116.2899, 95.9645) -> (-121.2898, 87.3045)
  arc A20 (-121.2898, 87.3045) -> (-122.2208, 83.4953) centre (-115.2277, 83.8044) ccw
  line L47 (-122.2208, 83.4953) -> (-125.0533, 51.1214)
  line L48 (-125.0533, 51.1214) -> (-127.1953, 51.3088)
  arc A21 (-127.1953, 51.3088) -> (-132.6119, 46.7636) centre (-127.6309, 46.3278) ccw
  line L49 (-132.6119, 46.7636) -> (-133.9192, 31.8207)
  arc A22 (-133.9192, 31.8207) -> (-129.374, 26.404) centre (-128.9383, 31.385) ccw
  line L50 (-129.374, 26.404) -> (-107.4576, 24.4867)
  line L51 (-107.4576, 24.4867) -> (-108.2856, 15.0227)
  arc A23 (-108.2856, 15.0227) -> (-106.6753, 9.9139) centre (-101.3122, 14.4126) ccw
  line L52 (-106.6753, 9.9139) -> (-106.2206, 9.3719)
  arc A24 (-106.2206, 9.3719) -> (-101.4678, 6.8976) centre (-100.8579, 13.871) ccw
  line L53 (-101.4678, 6.8976) -> (-89.2321, 5.8271)
  arc A25 (-89.2321, 5.8271) -> (-88.989, 5.5205) centre (-83.6277, 10.0212) ccw
  line L54 (-88.989, 5.5205) -> (-88.5345, 4.979)
  arc A26 (-88.5345, 4.979) -> (-83.7831, 2.5062) centre (-83.1731, 9.4796) ccw
  line L55 (-83.7831, 2.5062) -> (-67.513, 1.0828)
  arc A27 (-67.513, 1.0828) -> (-65.9211, -1.3752) centre (-60.9717, 3.5749) ccw
  line L56 (-65.9211, -1.3752) -> (-65.4205, -1.8756)
  arc A28 (-65.4205, -1.8756) -> (-60.4715, -3.925) centre (-60.4716, 3.075) ccw
  line L57 (-60.4715, -3.925) -> (-48.4717, -3.925)
  line L58 (-107.4576, 24.4867) -> (-107.109, 28.4715)
  line L59 (-129.9345, 31.4721) -> (-133.9192, 31.8207)
  constraint coincident L50.end L51.start
  constraint coincident L7 L58.end
  constraint perpendicular L7 L58
  constraint coincident A2.start L8.start
  constraint coincident L49.end A22.start
extrude "Extrude4" cut sketch "Sketch3" against normal blind 9 contours L7 A2 A22 L50 L58 L59 bodies 1
ref_plane "WorkPlane1" through (150, 0, 0) normal (1, 0, 0) x (0, 1, 0)
sketch "Sketch4" plane through (0, 0, 0) normal (0, 0, 1) x (1, 0, 0)
  line L0 (64.4695, 145.2633) -> (64.4695, 150.9263)
  line L1 (64.4695, 150.9263) -> (44.4711, 150.9263)
  line L2 (44.4711, 150.9263) -> (44.4711, 143.7003)
  arc A0 (44.0588, 143.5704) -> (44.4711, 143.7003) centre (43.9717, 144.5666) ccw
  line L3 (44.0588, 143.5704) -> (41.6085, 143.3561)
  line L4 (41.6085, 143.3561) -> (41.521, 144.3549)
  line L5 (41.521, 144.3549) -> (21.5989, 142.6108)
  line L6 (21.5989, 142.6108) -> (23.2539, 123.6817)
  line L7 (23.2539, 123.6817) -> (23.3283, 123.6882)
  arc A1 (22.9445, 123.4885) -> (23.3283, 123.6882) centre (22.6857, 124.4544) ccw
  line L8 (22.9445, 123.4885) -> (18.1064, 122.1922)
  line L9 (18.1064, 122.1922) -> (17.8471, 123.1603)
  line L10 (3.1869, 100.5974) -> (7.5863, 84.1761)
  line L11 (7.5863, 84.1761) -> (12.247, 66.7892)
  line L12 (31.5651, 71.9651) -> (27.7639, 86.1458)
  arc A2 (28.8143, 86.3799) -> (27.7639, 86.1458) centre (28.4724, 85.4401) ccw
  line L13 (28.8143, 86.3799) -> (77.0404, 68.827)
  line L14 (77.0404, 68.827) -> (76.6988, 67.8887)
  line L15 (76.6988, 67.8887) -> (94.5511, 61.3901)
  line L16 (94.5511, 61.3901) -> (111.0085, 51.8905)
  line L17 (111.0085, 51.8905) -> (120.5072, 68.3444)
  line L18 (120.5072, 68.3444) -> (118.4694, 69.5208)
  line L19 (103.6338, 121.9671) -> (105.1903, 139.766)
  line L20 (105.1903, 139.766) -> (87.2575, 141.3358)
  line L21 (87.2575, 141.3358) -> (87.5043, 144.1577)
  line L22 (87.5043, 144.1577) -> (67.5822, 145.9018)
  line L23 (67.5822, 145.9018) -> (67.4947, 144.9036)
  line L24 (67.4947, 144.9036) -> (64.8846, 145.1319)
  arc A3 (64.4695, 145.2633) -> (64.8846, 145.1319) centre (64.9717, 146.1281) ccw
  line L25 (61.4705, 134.4273) -> (61.4705, 148.4252)
  line L26 (70.3529, 143.1496) -> (69.1312, 129.2025)
  line L27 (47.4701, 114.4273) -> (47.4701, 100.4268)
  line L28 (6.4719, 99.9239) -> (10.0965, 86.4009)
  line L29 (61.4705, 114.4273) -> (47.4701, 114.4273)
  line L30 (100.5027, 120.602) -> (86.5556, 121.8212)
  line L31 (99.0194, 103.6679) -> (85.0722, 104.8871)
  line L32 (27.7673, 106.5101) -> (28.989, 92.563)
  line L33 (3.1869, 100.5974) -> (-1.4684, 117.9843)
  line L34 (12.247, 66.7892) -> (7.5863, 84.1761)
  line L35 (85.3338, 107.8766) -> (99.281, 106.6549)
  line L36 (81.5975, 111.0466) -> (82.8167, 124.9937)
  line L37 (2.0726, 116.345) -> (5.6972, 102.822)
  line L38 (80.3732, 69.2102) -> (93.5279, 64.4223)
  line L39 (61.4705, 100.4268) -> (61.4705, 114.4273)
  line L40 (10.8737, 83.5028) -> (14.4958, 69.9798)
  line L41 (23.6195, 90.0255) -> (19.9949, 103.5485)
  line L42 (42.9336, 93.7847) -> (41.7144, 107.7319)
  line L43 (99.281, 106.6549) -> (100.5027, 120.602)
  line L44 (28.0187, 73.6044) -> (24.3967, 87.1274)
  line L45 (82.8167, 124.9937) -> (68.8696, 126.2129)
  line L46 (15.5956, 119.967) -> (2.0726, 116.345)
  line L47 (47.4701, 117.427) -> (61.4705, 117.427)
  line L48 (-1.4684, 117.9843) -> (17.8471, 123.1603)
  line L49 (47.4701, 100.4268) -> (61.4705, 100.4268)
  line L50 (86.8172, 124.8108) -> (100.7643, 123.5916)
  line L51 (28.989, 92.563) -> (42.9336, 93.7847)
  line L52 (83.0783, 127.9833) -> (84.3001, 141.9279)
  line L53 (84.3001, 141.9279) -> (70.3529, 143.1496)
  line L54 (67.5822, 145.9018) -> (87.5043, 144.1577)
  line L55 (69.1312, 129.2025) -> (83.0783, 127.9833)
  line L56 (101.9835, 137.5362) -> (88.0364, 138.758)
  line L57 (19.9949, 103.5485) -> (6.4719, 99.9239)
  line L58 (61.4705, 131.4275) -> (47.4701, 131.4275)
  line L59 (41.4528, 110.7189) -> (40.2336, 124.666)
  line L60 (26.2865, 123.4468) -> (27.5057, 109.4997)
  line L61 (24.8056, 140.381) -> (26.0248, 126.4339)
  line L62 (24.3967, 87.1274) -> (10.8737, 83.5028)
  line L63 (19.2202, 106.4441) -> (15.5956, 119.967)
  line L64 (10.0965, 86.4009) -> (23.6195, 90.0255)
  line L65 (86.5556, 121.8212) -> (85.3338, 107.8766)
  line L66 (61.4705, 117.427) -> (61.4705, 131.4275)
  line L67 (44.4711, 150.9263) -> (64.4695, 150.9263)
  line L68 (47.4701, 131.4275) -> (47.4701, 117.427)
  line L69 (47.4701, 134.4273) -> (61.4705, 134.4273)
  line L70 (5.6972, 102.822) -> (19.2202, 106.4441)
  line L71 (61.4705, 148.4252) -> (47.4701, 148.4252)
  line L72 (14.4958, 69.9798) -> (28.0187, 73.6044)
  line L73 (31.5651, 71.9651) -> (12.247, 66.7892)
  line L74 (88.0364, 138.758) -> (86.8172, 124.8108)
  line L75 (100.7643, 123.5916) -> (101.9835, 137.5362)
  line L76 (68.8696, 126.2129) -> (67.6504, 112.2658)
  line L77 (39.972, 127.6556) -> (38.7502, 141.6028)
  line L78 (47.4701, 148.4252) -> (47.4701, 134.4273)
  line L79 (27.5057, 109.4997) -> (41.4528, 110.7189)
  line L80 (26.0248, 126.4339) -> (39.972, 127.6556)
  line L81 (38.7502, 141.6028) -> (24.8056, 140.381)
  line L82 (21.5989, 142.6108) -> (41.521, 144.3549)
  line L83 (41.7144, 107.7319) -> (27.7673, 106.5101)
  line L84 (40.2336, 124.666) -> (26.2865, 123.4468)
  line L85 (67.3887, 109.2787) -> (66.1695, 95.3316)
  line L86 (80.1141, 94.1124) -> (81.3359, 108.057)
  line L87 (85.0722, 104.8871) -> (83.853, 90.9399)
  line L88 (85.1611, 82.3674) -> (80.3732, 69.2102)
  line L89 (83.853, 90.9399) -> (97.8002, 89.7207)
  line L90 (109.6594, 55.5552) -> (116.6597, 67.6786)
  line L91 (97.536, 62.5554) -> (109.6594, 55.5552)
  line L92 (104.5337, 74.6788) -> (97.536, 62.5554)
  line L93 (93.5279, 64.4223) -> (98.3158, 77.5795)
  line L94 (81.3359, 108.057) -> (67.3887, 109.2787)
  line L95 (97.8002, 89.7207) -> (99.0194, 103.6679)
  arc A4 (94.8962, 62.3281) -> (95.0542, 62.2544) centre (94.5542, 61.3884) cw
  line L96 (116.6597, 67.6786) -> (104.5337, 74.6788)
  line L97 (120.5072, 68.3444) -> (111.0085, 51.8905)
  line L98 (98.3158, 77.5795) -> (85.1611, 82.3674)
  line L99 (66.1695, 95.3316) -> (80.1141, 94.1124)
  line L100 (67.6504, 112.2658) -> (81.5975, 111.0466)
  line L101 (118.4694, 69.5208) -> (99.981, 80.1945)
  line L102 (103.6338, 121.9671) -> (99.981, 80.1945)
  point P0 (0, 150)
  point P1 (27.7673, 106.5101)
  point P2 (24.8056, 140.381)
  point P3 (41.4528, 110.7189)
  point P4 (26.0248, 126.4339)
  point P5 (5.6972, 102.822)
  point P6 (6.4719, 99.9239)
  point P7 (61.4705, 148.4252)
  point P8 (61.4705, 131.4275)
  point P9 (15.5956, 119.967)
  point P10 (10.0965, 86.4009)
  point P11 (38.7502, 141.6028)
  point P12 (28.989, 92.563)
  point P13 (23.6195, 90.0255)
  point P14 (61.4705, 117.427)
  point P15 (39.972, 127.6556)
  point P16 (41.7144, 107.7319)
  point P17 (42.9336, 93.7847)
  point P18 (24.3967, 87.1274)
  point P19 (27.5057, 109.4997)
  point P20 (2.0726, 116.345)
  point P21 (47.4701, 131.4275)
  point P22 (40.2336, 124.666)
  point P23 (47.4701, 148.4252)
  point P24 (28.0187, 73.6044)
  point P25 (47.4701, 134.4273)
  point P26 (14.4958, 69.9798)
  point P27 (61.4705, 134.4273)
  point P28 (26.2865, 123.4468)
  point P29 (19.9949, 103.5485)
  point P30 (47.4701, 117.427)
  point P31 (19.2202, 106.4441)
  point P32 (10.8737, 83.5028)
  point P33 (83.853, 90.9399)
  point P34 (61.4705, 114.4273)
  point P35 (85.0722, 104.8871)
  point P36 (47.4701, 114.4273)
  point P37 (47.4701, 100.4268)
  point P38 (97.8002, 89.7207)
  point P39 (85.1611, 82.3674)
  point P40 (99.0194, 103.6679)
  point P41 (85.3338, 107.8766)
  point P42 (86.5556, 121.8212)
  point P43 (109.6594, 55.5552)
  point P44 (100.7643, 123.5916)
  point P45 (84.3001, 141.9279)
  point P46 (67.3887, 109.2787)
  point P47 (98.3158, 77.5795)
  point P48 (100.5027, 120.602)
  point P49 (80.3732, 69.2102)
  point P50 (82.8167, 124.9937)
  point P51 (80.1141, 94.1124)
  point P52 (86.8172, 124.8108)
  point P53 (101.9835, 137.5362)
  point P54 (68.8696, 126.2129)
  point P55 (99.281, 106.6549)
  point P56 (81.5975, 111.0466)
  point P57 (70.3529, 143.1496)
  point P58 (83.0783, 127.9833)
  point P59 (93.5279, 64.4223)
  point P60 (81.3359, 108.057)
  point P61 (104.5337, 74.6788)
  point P62 (97.536, 62.5554)
  point P63 (116.6597, 67.6786)
  point P64 (66.1695, 95.3316)
  point P65 (88.0364, 138.758)
  point P66 (69.1312, 129.2025)
  point P67 (61.4705, 100.4268)
  point P68 (67.6504, 112.2658)
  constraint coincident P20 L37.start
  constraint coincident P5 L37.end
  constraint coincident P31 L63.start
  constraint coincident P9 L46.start
  constraint parallel L37 L63
  constraint parallel L46 L70
  constraint coincident P6 L28.start
  constraint coincident P10 L28.end
  constraint parallel L28 L37
  constraint coincident P13 L41.start
  constraint perpendicular L28 L64
  constraint coincident P29 L41.end
  constraint parallel L28 L41
  constraint perpendicular L28 L57
  constraint coincident P32 L40.start
  constraint coincident P26 L40.end
  constraint coincident P24 L44.start
  constraint parallel L64 L72
  constraint coincident P18 L44.end
  constraint parallel L40 L44
  constraint coincident P1 L32.start
  constraint coincident P12 L32.end
  constraint coincident P17 L42.start
  constraint coincident P16 L42.end
  constraint perpendicular L32 L83
  constraint coincident P28 L60.start
  constraint coincident P19 L60.end
  constraint coincident P3 L59.start
  constraint coincident P22 L59.end
  constraint coincident P2 L61.start
  constraint coincident P4 L61.end
  constraint parallel L60 L61
  constraint coincident P15 L77.start
  constraint coincident P11 L77.end
  constraint perpendicular L77 L80
  constraint coincident P23 L71.end
  constraint coincident P25 L69.start
  constraint coincident P27 L25.start
  constraint perpendicular L69 L78
  constraint coincident P7 L25.end
  constraint perpendicular L25 L69
  constraint perpendicular L71 L78
  constraint coincident P21 L58.end
  constraint coincident P30 L47.start
  constraint coincident P14 L47.end
  constraint perpendicular L47 L68
  constraint coincident P8 L58.start
  constraint perpendicular L47 L66
  constraint perpendicular L58 L66
  constraint coincident P36 L27.start
  constraint coincident P37 L27.end
  constraint perpendicular L27 L47
  constraint coincident P67 L39.start
  constraint perpendicular L27 L49
  constraint coincident P34 L29.start
  constraint perpendicular L39 L47
  constraint perpendicular L27 L29
  constraint coincident P46 L85.start
  constraint coincident P64 L85.end
  constraint coincident P51 L86.start
  constraint coincident P60 L86.end
  constraint coincident P54 L45.end
  constraint coincident P68 L76.end
  constraint coincident P56 L36.start
  constraint perpendicular L76 L100
  constraint coincident P50 L36.end
  constraint perpendicular L36 L100
  constraint perpendicular L45 L76
  constraint coincident P57 L26.start
  constraint coincident P66 L26.end
  constraint coincident P58 L52.start
  constraint coincident P45 L52.end
  constraint coincident P65 L56.end
  constraint coincident P52 L50.start
  constraint coincident P44 L50.end
  constraint perpendicular L50 L74
  constraint coincident P53 L56.start
  constraint coincident P42 L30.end
  constraint coincident P41 L35.start
  constraint coincident P55 L35.end
  constraint parallel L35 L56
  constraint coincident P48 L30.start
  constraint perpendicular L35 L43
  constraint coincident P35 L31.end
  constraint coincident P33 L87.end
  constraint coincident P38 L89.end
  constraint perpendicular L87 L89
  constraint coincident L31.start L95.end
  constraint perpendicular L89 L95
  constraint perpendicular L31 L95
  constraint coincident P39 L88.start
  constraint coincident P49 L38.start
  constraint coincident P59 L38.end
  constraint coincident P47 L93.end
  constraint parallel L88 L93
  constraint parallel L38 L98
  constraint coincident P61 L92.start
  constraint coincident P62 L91.start
  constraint coincident P43 L90.start
  constraint coincident P63 L90.end
  constraint perpendicular L90 L91
  constraint parallel L18 L101
  constraint parallel L19 L102
extrude "Extrude5" add sketch "Sketch4" along normal blind 1.6 separate body makes body 2
sketch "Sketch5" plane through (0, 0, 0) normal (0, 0, 1) x (1, 0, 0)
  circle A0 centre (44.6674, -31.684) radius 1.25
  circle A1 centre (65.3052, -14.3667) radius 1.25
  circle A2 centre (61.9846, -52.3217) radius 1.25
  point P0 (46.8674, -31.684)
  point P1 (64.1846, -52.3217)
  point P2 (67.5052, -14.3667)
  point P3 (45.7674, -31.684)
  point P4 (63.0846, -52.3217)
  point P5 (66.4052, -14.3667)
  dimension "d33" = 2.5
  dimension "d34" = 2.5
  dimension "d35" = 2.5
  measures "d33" diameter of A0
  measures "d34" diameter of A1
  measures "d35" diameter of A2
move_body "Move1" bodies 2 to x (1, 0, 0) y (0, 1, 0) z (0, 0, 1) at (0, -150, 0)
extrude "Extrude6" cut sketch "Sketch5" along normal blind 2 and the other way blind 2 bodies 1 2
move_body "Move2" bodies 2 to x (1, 0, 0) y (0, 1, 0) z (0, 0, 1) at (0, 150, 0)
mirror "Mirror3" about plane through (150, 0, 0) normal (1, 0, 0) of bodies 1 2 makes body 3 at (206.159, -65.0404, -2) makes body 4 at (239.4252, 86.3541, 0)
